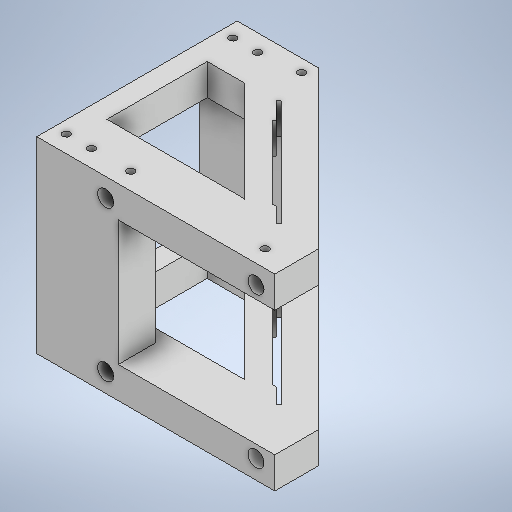
# Autodesk Inventor part: beamsplitter
Saved by Autodesk Inventor 2025.1 (Build 291241000, 241)
## iProperties
Created: 2024-11-22
Part Number: beamsplitter
Material: Ogólny
Document SubType Name: Modeling
Designer: PC
Density: 1 g/cm^3
Appearance: Domyślna
Author: PC
Autodesk Inventor part; units mm, degrees
ref_plane "YZ Plane" through (0, 0, 0) normal (1, 0, 0) x (0, 1, 0)
ref_plane "XZ Plane" through (0, 0, 0) normal (0, 1, 0) x (-1, 0, 0)
sketch "front" plane through (0, 0, 0) normal (0, 0, 1) x (1, 0, 0)
  line L0 (-30, 30) -> (30, 30) construction
  line L1 (30, 30) -> (30, -30) construction
  line L2 (30, -30) -> (-30, -30) construction
  line L3 (-30, -30) -> (-30, 30) construction
  line L4 (-30, 30) -> (30, -30) construction
  line L5 (30, 30) -> (-30, -30) construction
  circle A0 centre (-30, 30) radius 3.2
  circle A1 centre (30, 30) radius 3.2
  circle A2 centre (-30, -30) radius 3.2
  circle A3 centre (30, -30) radius 3.2
  line L6 (-37.5, 37.5) -> (37.5, 37.5)
  line L7 (37.5, 37.5) -> (37.5, -37.5)
  line L8 (37.5, -37.5) -> (-37.5, -37.5)
  line L9 (-37.5, -37.5) -> (-37.5, 37.5)
  line L10 (-37.5, 37.5) -> (37.5, -37.5) construction
  line L11 (37.5, 37.5) -> (-37.5, -37.5) construction
  line L12 (-25, -25) -> (25, -25)
  line L13 (25, -25) -> (25, 25)
  line L14 (25, 25) -> (-25, 25)
  line L15 (-25, 25) -> (-25, -25)
  line L16 (-25, -25) -> (25, 25) construction
  line L17 (25, -25) -> (-25, 25) construction
  point P0 (0, 0)
  dimension "d0" = 60
  dimension "d1" = 60
  dimension "d2" = 6.4
  dimension "d4" = 75
  dimension "d5" = 75
  dimension "d6" = 50
  dimension "d7" = 50
  constraints: 36 end point, 6 midpoint, 6 parallel, 4 centre point, 4 coincident, 3 equal radius, 3 horizontal, 3 perpendicular
  measures "d0" distance of L1.end L2.end
  measures "d1" distance of L0.end L1.end
  measures "d2" diameter of A0
  measures "d4" distance of L7.end L8.end
  measures "d5" distance of L6.end L7.end
  measures "d6" distance of L14.end L13.end
  measures "d7" distance of L13.end L12.end
extrude "main_shape" add sketch "front" against normal blind 80
sketch "gora" plane through (-37.5, 37.5, 0) normal (0, 1, 0) x (1, 0, 0)
  line L0 (70.7, 80) -> (70.7, 0) construction
  line L1 (64.3, 80) -> (64.3, 0) construction
  line L2 (10.7, 80) -> (10.7, 0) construction
  line L3 (4.3, 80) -> (4.3, 0) construction
  line L4 (75, 0) -> (75, 80) projected
  line L5 (0, 0) -> (0, 80) projected
  line L6 (0, 80) -> (75, 80) projected
  line L7 (75, 0) -> (0, 0) projected
  line L8 (75, 17.5) -> (12.5, 80)
  point P0 (37.5, 0)
  point P1 (62.5, 80)
  dimension "d19" = 45
  constraints: 2 end point, 2 point on line, 2 other
  measures "d19" angle of L4 L8
sketch "Szkic3" plane through (-37.5, -37.5, 0) normal (-1, 0, 0) x (0, 0, 1)
  line L0 (-80, 70.7) -> (0, 70.7) construction
  line L1 (-80, 64.3) -> (0, 64.3) construction
  line L2 (-80, 10.7) -> (0, 10.7) construction
  line L3 (-80, 4.3) -> (0, 4.3) construction
  line L4 (-80, 64.3) -> (-80, 70.7) construction
  line L5 (0, 70.7) -> (0, 64.3) construction
  line L6 (0, 10.7) -> (0, 4.3) construction
  line L7 (-80, 4.3) -> (-80, 10.7) construction
  circle A0 centre (-70, 67.5) radius 3.2
  circle A1 centre (-10, 67.5) radius 3.2
  circle A2 centre (-70, 7.5) radius 3.2
  circle A3 centre (-10, 7.5) radius 3.2
  point P0 (0, 37.5)
  dimension "d10" = 6.4
  dimension "d11" = 6.4
  dimension "d12" = 6.4
  dimension "d13" = 6.4
  dimension "d14" = 60
  dimension "d15" = 10
  constraints: 4 centre point, 2 vertical alignment
  measures "d10" diameter of A0
  measures "d11" diameter of A1
  measures "d12" diameter of A2
  measures "d13" diameter of A3
  measures "d14" distance of A1.centre A0.centre
  measures "d15" distance from line of L4 A0.centre
extrude "Wyciągnięcie proste2" cut sketch "gora" against normal through all contours L8 L6 L4
extrude "Otwory prostopadle" cut sketch "Szkic3" against normal blind 5
sketch "Szkic5" plane through (-37.5, -37.5, 0) normal (-1, 0, 0) x (0, 0, 1)
  circle A0 centre (-70, 67.5) radius 3.2 construction
  circle A1 centre (-10, 67.5) radius 3.2 construction
  circle A2 centre (-10, 7.5) radius 3.2 construction
  circle A3 centre (-70, 7.5) radius 3.2 construction
  line L0 (-70, 67.5) -> (-10, 67.5) construction
  line L1 (-10, 67.5) -> (-10, 7.5) construction
  line L2 (-65, 12.5) -> (-15, 12.5)
  line L3 (-15, 12.5) -> (-15, 62.5)
  line L4 (-15, 62.5) -> (-65, 62.5)
  line L5 (-65, 62.5) -> (-65, 12.5)
  line L6 (-65, 12.5) -> (-15, 62.5) construction
  line L7 (-15, 12.5) -> (-65, 62.5) construction
  point P0 (0, 37.5)
  point P1 (-40, 37.5)
  point P2 (-40, 67.5)
  point P3 (-10, 37.5)
  dimension "d27" = 50
  dimension "d28" = 50
  constraints: 16 end point, 4 midpoint, 2 horizontal, 2 parallel, 2 perpendicular, 1 horizontal alignment, 1 vertical alignment
  measures "d27" distance of L4.end L3.end
  measures "d28" distance of L3.end L2.end
extrude "Wyciągnięcie proste5" cut sketch "Szkic5" against normal through all
sketch "Szkic4" plane through (-37.5, 37.5, 0) normal (0, 1, 0) x (1, 0, 0)
  line L0 (0, 66.8) -> (0, 73.2) construction
  line L1 (4.3, 80) -> (10.7, 80) construction
  line L2 (0, 6.8) -> (0, 13.2) construction
  line L3 (10.7, 0) -> (4.3, 0) construction
  line L4 (70.7, 0) -> (64.3, 0) construction
  line L5 (7.5, 80) -> (7.5, 0) construction
  line L6 (0, 10) -> (75, 10) construction
  line L7 (0, 70) -> (7.5, 70) construction
  line L8 (7.5, 70) -> (75.5272, 1.9728) construction
  line L9 (10.7, 80) -> (10.7, 0) construction
  line L10 (10.7, 80) -> (10.7, 0) construction
  line L11 (4.3, 80) -> (4.3, 0) construction
  line L12 (64.3, 28.2) -> (64.3, 0) construction
  line L13 (70.7, 21.8) -> (70.7, 0) construction
  line L14 (12.5, 0) -> (12.5, 80) construction
  line L15 (12.5, 80) -> (12.5, 0) construction
  line L16 (12.5, 0) -> (62.5, 0) construction
  line L17 (62.5, 30) -> (62.5, 0) construction
  line L18 (16.2868, 61.2132) -> (58.7132, 18.7868)
  line L19 (75, 0) -> (0, 0) projected
  line L20 (15.2968, 60.2233) -> (57.7233, 17.7968)
  line L21 (15.2968, 60.2233) -> (16.2868, 61.2132)
  line L22 (57.7233, 17.7968) -> (58.7132, 18.7868)
  line L23 (16.2868, 61.2132) -> (12.5, 65)
  line L24 (12.5, 80) -> (12.5, 65)
  line L25 (0, 0) -> (0, 80) projected
  line L26 (12.5, 80) -> (62.5, 30)
  line L27 (58.7132, 18.7868) -> (62.5, 15)
  line L28 (62.5, 30) -> (62.5, 15)
  point P0 (37.5, 0)
  point P1 (37.5, 40)
  point P2 (37.5, 0)
  dimension "d22" = 45
  dimension "d23" = 60
  dimension "d24" = 1.4
  constraints: 30 end point, 6 midpoint, 6 point on line, 3 perpendicular, 2 collinear, 2 parallel, 1 vertical, 1 vertical alignment, 2 other
  measures "d22" angle of L5 L8
  measures "d23" distance of L18.start L18.end
  measures "d24" distance between parallel lines of L18 L20
extrude "Wyciągnięcie proste4" cut sketch "Szkic4" against normal blind 70 contours L18 L22 L20 L21
sketch "Szkic6" plane through (-37.5, -37.5, 0) normal (-1, 0, 0) x (0, 0, 1)
  line L0 (-65, 62.5) -> (-15, 62.5) projected
  line L1 (-15, 62.5) -> (-15, 12.5) projected
  line L2 (-15, 12.5) -> (-65, 12.5) projected
  line L3 (-65, 12.5) -> (-65, 62.5) projected
  circle A0 centre (-10, 7.5) radius 3.2 projected
  circle A1 centre (-10, 67.5) radius 3.2 projected
  circle A2 centre (-70, 7.5) radius 3.2 projected
  circle A3 centre (-70, 67.5) radius 3.2 projected
  line L4 (0, 75) -> (0, 0) projected
  line L5 (0, 75) -> (-80, 75) projected
  line L6 (-80, 0) -> (-80, 75) projected
  line L7 (0, 0) -> (-80, 0) projected
  point P0 (0, 37.5)
extrude "prowadnice prostopadle" add sketch "Szkic6" along normal blind 20
sketch "Szkic7" plane through (0, 0, 0) normal (0, 0, 1) x (1, 0, 0)
  line L0 (25, 25) -> (25, -25) projected
  line L1 (37.5, -37.5) -> (37.5, 37.5) projected
  line L2 (21.2132, 25) -> (-21.2132, 25) projected
  line L3 (-21.2132, 25) -> (-22.2032, 25) projected
  line L4 (-22.2032, 25) -> (20.2233, 25) projected
  line L5 (20.2233, 25) -> (21.2132, 25) projected
  line L6 (-25, 25) -> (25, 25) projected
  line L7 (-25, 25) -> (-57.5, 25) projected
  line L8 (-57.5, 25) -> (-25, 25) projected
  line L9 (-25, 25) -> (37.5, 25) projected
  line L10 (25, 25) -> (37.5, 25) projected
  line L11 (-21.2132, -25) -> (21.2132, -25) projected
  line L12 (21.2132, -25) -> (20.2233, -25) projected
  line L13 (20.2233, -25) -> (-22.2032, -25) projected
  line L14 (-22.2032, -25) -> (-21.2132, -25) projected
  line L15 (25, -25) -> (-25, -25) projected
  line L16 (25, -25) -> (37.5, -25) projected
  line L17 (37.5, -25) -> (-25, -25) projected
  line L18 (-57.5, -25) -> (-25, -25) projected
  line L19 (-57.5, -25) -> (-25, -25) projected
  point P0 (0, 0)
extrude "Wyciągnięcie proste7" cut sketch "Szkic7" against normal through all
sketch "Szkic8" plane through (37.5, 37.5, 0) normal (0, 1, 0) x (1, 0, 0)
  line L0 (-64.3, 80) -> (-64.3, 0) construction
  line L1 (-70.7, 80) -> (-70.7, 0) construction
  line L2 (-4.3, 21.8) -> (-4.3, 0) construction
  line L3 (-10.7, 28.2) -> (-10.7, 0) construction
  line L4 (-95, 6.8) -> (-70.7, 6.8) construction
  line L5 (-95, 13.2) -> (-70.7, 13.2) construction
  line L6 (-95, 66.8) -> (-70.7, 66.8) construction
  line L7 (-95, 66.8) -> (-70.7, 66.8) construction
  line L8 (-95, 73.2) -> (-70.7, 73.2) construction
  circle A0 centre (-90, 6.8) radius 1.5
  circle A1 centre (-80, 6.8) radius 1.5
  circle A2 centre (-90, 73.2) radius 1.5
  circle A3 centre (-80, 73.2) radius 1.5
  circle A4 centre (-64.3, 75) radius 1.5
  circle A5 centre (-64.3, 6.8) radius 1.5
  line L9 (0, 0) -> (-95, 0) projected
  line L10 (-95, 0) -> (-95, 80) projected
  line L11 (-62.5, 80) -> (-95, 80) projected
  circle A6 centre (-10.7, 6.8) radius 1.5
  point P0 (-37.5, 0)
  dimension "d35" = 3
  dimension "d36" = 3
  dimension "d37" = 3
  dimension "d38" = 3
  dimension "d39" = 10
  dimension "d40" = 3
  dimension "d41" = 3
  dimension "d44" = 5
  dimension "d45" = 5
  dimension "d46" = 3
  constraints: 7 centre point, 5 point on line, 4 horizontal alignment, 2 vertical alignment
  measures "d35" diameter of A0
  measures "d36" diameter of A1
  measures "d37" diameter of A2
  measures "d38" diameter of A3
  measures "d39" distance of A0.centre A1.centre
  measures "d40" diameter of A4
  measures "d41" diameter of A5
  measures "d44" distance from line of L10 A0.centre
  measures "d45" distance from line of L11 A4.centre
  measures "d46" diameter of A6
extrude "robaczki" cut sketch "Szkic8" against normal blind 10
ref_plane "Płaszczyzna konstrukcyjna2" through (37.5, 0, 0) normal (0, 1, 0) x (1, 0, 0)
mirror "Odbij1" about plane through (37.5, 0, 0) normal (0, 1, 0) of "robaczki"
sketch "Szkic9" plane through (37.5, 37.5, 0) normal (0, 1, 0) x (1, 0, 0)
  line L0 (0, 17.5) -> (-62.5, 80) construction
  line L1 (-62.5, 65) -> (-62.5, 80) construction
  line L2 (-95, 65) -> (-62.5, 65) construction
  line L3 (-95, 15) -> (-95, 65) construction
  line L4 (-95, 15) -> (-62.5, 15) construction
  line L5 (-62.5, 0) -> (-62.5, 15) construction
  line L6 (0, 0) -> (-62.5, 0) construction
  line L7 (0, 17.5) -> (0, 0) construction
  line L8 (-58.7132, 61.2132) -> (-16.2868, 18.7868) construction
  line L9 (-16.2868, 18.7868) -> (-17.2767, 17.7968) construction
  line L10 (-17.2767, 17.7968) -> (-59.7032, 60.2233) construction
  line L11 (-59.7032, 60.2233) -> (-58.7132, 61.2132) construction
  line L12 (-87, 60) -> (-72, 60)
  line L13 (-72, 60) -> (-32, 20)
  line L14 (-32, 20) -> (-87, 20)
  line L15 (-87, 20) -> (-87, 60)
  line L16 (-17.2767, 17.7968) -> (-59.7032, 60.2233) construction
  point P0 (-37.5, 0)
  dimension "d49" = 8
  dimension "d50" = 5
  dimension "d51" = 5
  dimension "d52" = 55
  constraints: 8 end point, 2 parallel, 1 horizontal, 1 perpendicular
  measures "d49" distance between parallel lines of L15 L3
  measures "d50" distance between parallel lines of L4 L14
  measures "d51" distance between parallel lines of L2 L12
  measures "d52" distance of L14.end L13.end
extrude "Wyciągnięcie proste9" cut sketch "Szkic9" against normal through all
sketch "Szkic10" plane through (37.5, -37.5, -17.5) normal (0.7071, 0, -0.7071) x (-0.7071, 0, -0.7071)
  line L0 (12.4264, 12.5) -> (72.4264, 12.5) projected
  line L1 (12.4264, 12.5) -> (12.4264, 5) projected
  line L2 (12.4264, 5) -> (72.4264, 5) projected
  line L3 (72.4264, 12.5) -> (72.4264, 5) projected
  line L4 (72.4264, 62.5) -> (12.4264, 62.5) projected
  line L5 (72.4264, 75) -> (72.4264, 62.5) projected
  line L6 (12.4264, 75) -> (72.4264, 75) projected
  line L7 (12.4264, 75) -> (12.4264, 62.5) projected
  circle A0 centre (17.4264, 70) radius 1.5
  circle A1 centre (67.4264, 70) radius 1.5
  circle A2 centre (67.4264, 7.5) radius 1.5
  circle A3 centre (17.4264, 7.5) radius 1.5
  point P0 (14.1421, 37.5)
  dimension "d55" = 3
  dimension "d56" = 5
  dimension "d57" = 5
  dimension "d60" = 5
  dimension "d61" = 5
  constraints: 4 centre point, 3 equal radius, 2 horizontal alignment, 2 vertical alignment
  measures "d55" diameter of A0
  measures "d56" distance from line of L6 A0.centre
  measures "d57" distance from line of L0 A3.centre
  measures "d60" horizontal distance of L6.start A0.centre
  measures "d61" horizontal distance of L5.start A1.centre
extrude "Wyciągnięcie proste10" cut sketch "Szkic10" against normal up to surface (12.0066 mm away) contours A0 | A1 | A2 | A3
sketch "Szkic11" plane through (37.5, 37.5, 0) normal (0, 1, 0) x (1, 0, 0)
  line L0 (-59.7032, 60.2233) -> (-17.2767, 17.7968) construction
  line L1 (-17.2767, 17.7968) -> (-59.7032, 60.2233) construction
  line L2 (-48.7383, 66.2383) -> (-46.617, 64.117) construction
  line L3 (-13.383, 30.883) -> (-11.2617, 28.7617) construction
  line L4 (-13.383, 30.883) -> (-20.883, 23.383) construction
  line L5 (-11.2617, 28.7617) -> (-18.7617, 21.2617) construction
  line L6 (-48.7383, 66.2383) -> (-56.2383, 58.7383) construction
  line L7 (-46.617, 64.117) -> (-54.117, 56.617) construction
  line L8 (-58.7132, 61.2132) -> (-16.2868, 18.7868) projected
  line L9 (-59.7032, 60.2233) -> (-58.7132, 61.2132) projected
  line L10 (-17.2767, 17.7968) -> (-59.7032, 60.2233) projected
  line L11 (-16.2868, 18.7868) -> (-17.2767, 17.7968) projected
  line L12 (-52.9856, 53.5057) -> (-53.6927, 52.7986)
  line L13 (-70.7, 58.7) -> (-64.3, 52.3) projected
  line L14 (-53.6927, 52.7986) -> (-24.7014, 23.8073)
  line L15 (-24.7014, 23.8073) -> (-23.2872, 23.8073)
  point P0 (-37.5, 0)
  point P1 (-23.9943, 24.5144)
  dimension "d62" = 3
  dimension "d63" = 3
  dimension "d64" = 1
  constraints: 6 end point, 3 point on line, 1 horizontal, 1 parallel, 1 perpendicular
  measures "d62" distance from line of L4 L14.end
  measures "d63" distance between parallel lines of L7 L12
  measures "d64" distance between parallel lines of L0 L14
extrude "Wyciągnięcie proste11" cut sketch "Szkic11" against normal through all
sketch "Szkic12" plane through (-57.5, -37.5, 0) normal (-1, 0, 0) x (0, 0, 1)
  circle A0 centre (-33.342, -2.992) radius 2.25
  line L0 (-16.658, -6.908) -> (-50.026, -6.908)
  line L1 (-50.026, -6.908) -> (-50.026, 0)
  line L2 (-50.026, 0) -> (-16.658, 0)
  line L3 (-16.658, 0) -> (-16.658, -6.908)
  line L4 (-48.1515, 0) -> (-48.1515, 75.5094) construction
  line L5 (-20, 75) -> (-60, 75) construction
  line L6 (0, 37.5) -> (-80, 37.5) construction
  line L7 (-80, 62.5) -> (-80, 12.5) construction
  line L8 (-16.658, 0) -> (-50.026, 0) construction
  circle A1 centre (-62.961, -2.992) radius 2.25
  line L9 (-79.645, -6.908) -> (-46.277, -6.908)
  line L10 (-46.277, -6.908) -> (-46.277, 0)
  line L11 (-46.277, 0) -> (-79.645, 0)
  line L12 (-79.645, 0) -> (-79.645, -6.908)
  circle A2 centre (-33.342, 77.992) radius 2.25
  line L13 (-16.658, 81.908) -> (-50.026, 81.908)
  line L14 (-50.026, 81.908) -> (-50.026, 75)
  line L15 (-50.026, 75) -> (-16.658, 75)
  line L16 (-16.658, 75) -> (-16.658, 81.908)
  line L17 (-16.658, 75) -> (-50.026, 75) construction
  circle A3 centre (-62.961, 77.992) radius 2.25
  line L18 (-46.277, 81.908) -> (-46.277, 75)
  line L19 (-79.645, 81.908) -> (-46.277, 81.908)
  line L20 (-79.645, 75) -> (-79.645, 81.908)
  line L21 (-46.277, 75) -> (-79.645, 75)
  line L22 (-80, 0) -> (0, 0) construction
  point P0 (-48.1515, 75)
  point P1 (-33.342, 0)
  point P2 (-33.342, 0)
  dimension "d67" = 4.5
  dimension "d68" = 2.992
  dimension "d69" = 6.908
  dimension "d70" = 29.619
  dimension "d71" = 16.684
  dimension "d74" = 17.039
  constraints: 40 end point, 16 symmetric about line, 4 centre point, 3 midpoint, 3 perpendicular, 2 parallel, 1 collinear, 1 horizontal, 1 horizontal alignment, 1 vertical alignment, 3 other
  measures "d67" diameter of A0
  measures "d68" distance of point (-33.342, 0) A0.centre
  measures "d69" distance between parallel lines of L2 L0
  measures "d70" distance of A1.centre A0.centre
  measures "d71" distance from line of A0.centre L3
  measures "d74" horizontal distance of L22.start A1.centre
extrude "Wyciągnięcie proste12" [suppressed]
sketch "Szkic13" plane through (-49.5, 25, -60) normal (1, 0, 0) x (0, 0, -1)
  circle A0 centre (-31, -65) radius 2.25 projected
  circle A1 centre (-31, -65) radius 4
  circle A2 centre (4, -65) radius 2.25 projected
  circle A3 centre (4, -65) radius 4
  circle A4 centre (4, 15) radius 2.25 projected
  circle A5 centre (4, 15) radius 4
  circle A6 centre (-31, 15) radius 2.25 projected
  circle A7 centre (-31, 15) radius 4
  point P0 (-60, -25)
  dimension "d75" = 8
  dimension "d76" = 8
  dimension "d77" = 8
  dimension "d78" = 8
  constraints: 4 centre point, 4 coincident
  measures "d75" diameter of A1
  measures "d76" diameter of A3
  measures "d77" diameter of A5
  measures "d78" diameter of A7
extrude "Wyciągnięcie proste13" [suppressed]
ref_plane "Płaszczyzna konstrukcyjna3" through (37.5, 0, 0) normal (0, 1, 0) x (1, 0, 0)
